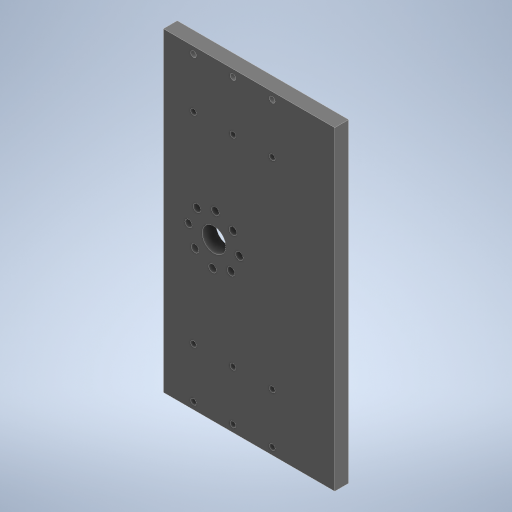
# Autodesk Inventor part: 12
Saved by Autodesk Inventor 2024.3 (Build 283343000, 343)
## iProperties
Created: 2024-09-08
Part Number: 12
Material: 아크릴, 선명
Document SubType Name: Modeling
Designer: 구지현
Density: 1.19 g/cm^3
Appearance: 회색
Mass: 66.4726 g
Surface Area: 217.278 cm^2
Volume: 55.8594 cm^3
Author: 구지현
Autodesk Inventor part; units mm, degrees
ref_plane "YZ Plane" through (0, 0, 0) normal (1, 0, 0) x (0, 1, 0)
ref_plane "XZ Plane" through (0, 0, 0) normal (0, 1, 0) x (-1, 0, 0)
ref_plane "XY Plane" through (0, 0, 0) normal (0, 0, 1) x (1, 0, 0)
ref_plane "작업 평면1" through (-11.501, -90.6951, 25.5) normal (0, 0, 1) x (0, 1, 0)
sketch "스케치1" plane through (-11.501, -90.6951, 25.5) normal (0, 0, 1) x (0, 1, 0)
  line L0 (-0.0049, 0) -> (27.5951, 0) projected
  line L1 (27.5951, 0) -> (27.5951, 6) projected
  line L2 (-0.0049, 6) -> (27.5951, 6) projected
  line L3 (-0.0049, 0) -> (-0.0049, 6) projected
  line L4 (127.3951, 6) -> (99.7951, 6) projected
  line L5 (99.7951, 6) -> (99.7951, 0) projected
  line L6 (127.3951, 0) -> (99.7951, 0) projected
  line L7 (127.3951, 6) -> (127.3951, 0) projected
  line L8 (99.8951, -54.101) -> (127.4951, -54.101) projected
  line L9 (127.4951, -54.101) -> (127.4951, -48.101) projected
  line L10 (99.8951, -48.101) -> (127.4951, -48.101) projected
  line L11 (99.8951, -54.101) -> (99.8951, -48.101) projected
  line L12 (27.4951, -48.101) -> (-0.1049, -48.101) projected
  line L13 (-0.1049, -48.101) -> (-0.1049, -54.101) projected
  line L14 (27.4951, -54.101) -> (-0.1049, -54.101) projected
  line L15 (27.4951, -48.101) -> (27.4951, -54.101) projected
  line L16 (-0.2463, -60.601) -> (-0.2463, -62.601) projected
  line L17 (-0.2463, -62.601) -> (1.1951, -62.601) projected
  line L18 (1.1951, -62.601) -> (1.1951, -92.601) projected
  line L19 (1.1951, -92.601) -> (-0.2463, -92.601) projected
  line L20 (-0.2463, -92.601) -> (-0.2463, -94.601) projected
  line L21 (-0.2463, -94.601) -> (6.0451, -94.601) projected
  line L22 (21.3451, -94.601) -> (6.0451, -94.601) projected
  line L23 (21.3451, -94.601) -> (27.6365, -94.601) projected
  line L24 (27.6365, -92.601) -> (27.6365, -94.601) projected
  line L25 (27.6365, -92.601) -> (26.1951, -92.601) projected
  line L26 (26.1951, -62.601) -> (26.1951, -92.601) projected
  line L27 (26.1951, -62.601) -> (27.6365, -62.601) projected
  line L28 (27.6365, -60.601) -> (27.6365, -62.601) projected
  line L29 (27.6365, -60.601) -> (26.6951, -60.601) projected
  line L30 (26.6951, -60.601) -> (26.6951, -59.101) projected
  line L31 (0.6951, -59.101) -> (26.6951, -59.101) projected
  line L32 (0.6951, -59.101) -> (0.6951, -60.601) projected
  line L33 (0.6951, -60.601) -> (-0.2463, -60.601) projected
  line L34 (35.6951, -14.501) -> (35.6951, -37.501) projected
  line L35 (35.6951, -14.501) -> (30.6951, -14.501) projected
  line L36 (30.6951, -14.501) -> (30.6951, -11.001) projected
  line L37 (28.6951, -11.001) -> (30.6951, -11.001) projected
  line L38 (28.6951, -11.001) -> (28.6951, -13.501) projected
  line L39 (28.6951, -13.501) -> (-1.3049, -13.501) projected
  line L40 (-1.3049, -13.501) -> (-1.3049, -11.001) projected
  line L41 (-1.3049, -11.001) -> (-3.3049, -11.001) projected
  line L42 (-3.3049, -11.001) -> (-3.3049, -16.751) projected
  line L43 (-5.8049, -16.751) -> (-3.3049, -16.751) projected
  spline S0 degree 3 poles (-5.8049, -16.751) (-6.0293, -16.751) (-6.2964, -16.7855) (-6.6655, -16.908) (-6.8416, -16.9972) (-7.0685, -17.1834) (-7.1685, -17.3017) (-7.2736, -17.5152) (-7.3049, -17.6421) (-7.3049, -17.751) knots -0.188065 -0.188065 -0.188065 -0.188065 -0.120738 -0.120738 -0.071394 -0.071394 -0.032672 -0.032672 0 0 0 0 projected
  line L44 (-7.3049, -34.251) -> (-7.3049, -17.751) projected
  spline S1 degree 3 poles (-7.3049, -34.251) (-7.3049, -34.3599) (-7.2736, -34.4868) (-7.1685, -34.7003) (-7.0685, -34.8186) (-6.8416, -35.0048) (-6.6655, -35.094) (-6.2964, -35.2165) (-6.0293, -35.251) (-5.8049, -35.251) knots 0 0 0 0 0.032672 0.032672 0.071394 0.071394 0.120738 0.120738 0.188065 0.188065 0.188065 0.188065 projected
  line L45 (-5.8049, -35.251) -> (-3.3049, -35.251) projected
  line L46 (-3.3049, -35.251) -> (-3.3049, -41.001) projected
  line L47 (-1.3049, -41.001) -> (-3.3049, -41.001) projected
  line L48 (-1.3049, -41.001) -> (-1.3049, -38.501) projected
  line L49 (28.6951, -38.501) -> (-1.3049, -38.501) projected
  line L50 (28.6951, -38.501) -> (28.6951, -41.001) projected
  line L51 (28.6951, -41.001) -> (30.6951, -41.001) projected
  line L52 (30.6951, -41.001) -> (30.6951, -37.501) projected
  line L53 (35.6951, -37.501) -> (30.6951, -37.501) projected
  line L54 (135.6951, -14.501) -> (135.6951, -37.501) projected
  line L55 (135.6951, -14.501) -> (130.6951, -14.501) projected
  line L56 (130.6951, -14.501) -> (130.6951, -11.001) projected
  line L57 (128.6951, -11.001) -> (130.6951, -11.001) projected
  line L58 (128.6951, -11.001) -> (128.6951, -13.501) projected
  line L59 (128.6951, -13.501) -> (98.6951, -13.501) projected
  line L60 (98.6951, -13.501) -> (98.6951, -11.001) projected
  line L61 (98.6951, -11.001) -> (96.6951, -11.001) projected
  line L62 (96.6951, -11.001) -> (96.6951, -16.751) projected
  line L63 (94.1951, -16.751) -> (96.6951, -16.751) projected
  spline S2 degree 3 poles (94.1951, -16.751) (93.9707, -16.751) (93.7036, -16.7855) (93.3345, -16.908) (93.1584, -16.9972) (92.9315, -17.1834) (92.8315, -17.3017) (92.7264, -17.5152) (92.6951, -17.6421) (92.6951, -17.751) knots -0.188065 -0.188065 -0.188065 -0.188065 -0.120738 -0.120738 -0.071394 -0.071394 -0.032672 -0.032672 0 0 0 0 projected
  line L64 (92.6951, -34.251) -> (92.6951, -17.751) projected
  spline S3 degree 3 poles (92.6951, -34.251) (92.6951, -34.3599) (92.7264, -34.4868) (92.8315, -34.7003) (92.9315, -34.8186) (93.1584, -35.0048) (93.3345, -35.094) (93.7036, -35.2165) (93.9707, -35.251) (94.1951, -35.251) knots 0 0 0 0 0.032672 0.032672 0.071394 0.071394 0.120738 0.120738 0.188065 0.188065 0.188065 0.188065 projected
  line L65 (94.1951, -35.251) -> (96.6951, -35.251) projected
  line L66 (96.6951, -35.251) -> (96.6951, -41.001) projected
  line L67 (98.6951, -41.001) -> (96.6951, -41.001) projected
  line L68 (98.6951, -41.001) -> (98.6951, -38.501) projected
  line L69 (128.6951, -38.501) -> (98.6951, -38.501) projected
  line L70 (128.6951, -38.501) -> (128.6951, -41.001) projected
  line L71 (128.6951, -41.001) -> (130.6951, -41.001) projected
  line L72 (130.6951, -41.001) -> (130.6951, -37.501) projected
  line L73 (135.6951, -37.501) -> (130.6951, -37.501) projected
  line L74 (99.7537, -60.601) -> (99.7537, -62.601) projected
  line L75 (99.7537, -62.601) -> (101.1951, -62.601) projected
  line L76 (101.1951, -62.601) -> (101.1951, -92.601) projected
  line L77 (101.1951, -92.601) -> (99.7537, -92.601) projected
  line L78 (99.7537, -92.601) -> (99.7537, -94.601) projected
  line L79 (99.7537, -94.601) -> (106.0451, -94.601) projected
  line L80 (121.3451, -94.601) -> (106.0451, -94.601) projected
  line L81 (121.3451, -94.601) -> (127.6365, -94.601) projected
  line L82 (127.6365, -92.601) -> (127.6365, -94.601) projected
  line L83 (127.6365, -92.601) -> (126.1951, -92.601) projected
  line L84 (126.1951, -62.601) -> (126.1951, -92.601) projected
  line L85 (126.1951, -62.601) -> (127.6365, -62.601) projected
  line L86 (127.6365, -60.601) -> (127.6365, -62.601) projected
  line L87 (127.6365, -60.601) -> (126.6951, -60.601) projected
  line L88 (126.6951, -60.601) -> (126.6951, -59.101) projected
  line L89 (100.6951, -59.101) -> (126.6951, -59.101) projected
  line L90 (100.6951, -59.101) -> (100.6951, -60.601) projected
  line L91 (100.6951, -60.601) -> (99.7537, -60.601) projected
  line L92 (21.3451, 6) -> (21.3451, 12)
  line L93 (1.1951, -62.601) -> (1.1951, 11.399)
  line L94 (-24.3049, -26.001) -> (-24.3049, -76.001) projected
  line L95 (-24.3049, -76.001) -> (-18.3049, -76.001) projected
  line L96 (-18.3049, -26.001) -> (-18.3049, -76.001) projected
  line L97 (-24.3049, -26.001) -> (-18.3049, -26.001) projected
  line L98 (145.6951, -26.001) -> (145.6951, -76.001) projected
  line L99 (145.6951, -76.001) -> (151.6951, -76.001) projected
  line L100 (151.6951, -26.001) -> (151.6951, -76.001) projected
  line L101 (145.6951, -26.001) -> (151.6951, -26.001) projected
  line L102 (-24.3049, -52.5323) -> (151.6951, -52.5323)
  line L103 (1.1951, 11.399) -> (-33.5056, 11.399)
  line L104 (1.1951, -62.601) -> (-24.3049, -62.601)
  line L105 (-24.3049, -62.601) -> (151.6951, -62.601)
  line L106 (151.6951, -62.601) -> (151.6951, 11.399)
  line L107 (151.6951, 11.399) -> (-24.3049, 11.399)
  line L108 (-24.3049, 11.399) -> (-24.3049, -62.601)
  circle A0 centre (-0.0049, 0) radius 1
  circle A1 centre (-0.0049, 6) radius 1
  circle A2 centre (27.5951, 6) radius 1
  circle A3 centre (27.5951, 0) radius 1
  circle A4 centre (99.7951, 0) radius 1
  circle A5 centre (99.7951, 6) radius 1
  circle A6 centre (127.3951, 6) radius 1
  circle A7 centre (127.3951, 0) radius 1
  circle A8 centre (99.8951, -54.101) radius 1
  circle A9 centre (99.8951, -48.101) radius 1
  circle A10 centre (127.4951, -48.101) radius 1
  circle A11 centre (127.6365, -54.101) radius 1
  circle A12 centre (27.4951, -54.101) radius 1
  circle A13 centre (27.5951, -48.101) radius 1
  circle A14 centre (-0.1049, -48.101) radius 1
  circle A15 centre (-0.1049, -54.101) radius 1
  point P0 (90.6951, -11.501)
  point P1 (99.8951, -49.101)
  point P2 (100.8951, -48.101)
  point P3 (126.4951, -48.101)
  point P4 (127.4951, -49.101)
  point P5 (127.4951, -53.1111)
  point P6 (126.6365, -54.101)
  point P7 (100.8951, -54.101)
  point P8 (99.8951, -53.101)
  point P9 (126.3951, 0)
  point P10 (100.7951, 0)
  point P11 (99.7951, 1)
  point P12 (99.7951, 5)
  point P13 (100.7951, 6)
  point P14 (126.3951, 6)
  point P15 (127.3951, 5)
  point P16 (127.3951, 1)
  point P17 (26.5951, 6)
  point P18 (27.5951, 5)
  point P19 (27.5951, 1)
  point P20 (26.5951, 0)
  point P21 (0.9951, 0)
  point P22 (-0.0049, 1)
  point P23 (-0.0049, 5)
  point P24 (0.9951, 6)
  point P25 (26.5951, -48.101)
  point P26 (27.4951, -49.096)
  point P27 (27.4951, -53.101)
  point P28 (26.4951, -54.101)
  point P29 (0.8951, -54.101)
  point P30 (-0.1049, -53.101)
  point P31 (-0.1049, -49.101)
  point P32 (0.8951, -48.101)
  point P33 (-0.2463, -62.601)
  point P34 (1.1951, -62.601)
  point P35 (99.7537, -62.601)
  point P36 (101.1951, -62.601)
  point P37 (126.1951, -62.601)
  point P38 (127.6365, -62.601)
  point P39 (151.6951, -62.601)
  point P40 (1.1951, 11.399)
  point P41 (-24.3049, 11.399)
  dimension "d0" = 6
  dimension "d1" = 74
  dimension "d2" = 2
  dimension "d3" = 2
  dimension "d4" = 2
  dimension "d5" = 2
  dimension "d6" = 2
  dimension "d7" = 2
  dimension "d8" = 2
  dimension "d9" = 2
  dimension "d10" = 2
  dimension "d11" = 2
  dimension "d12" = 2
  dimension "d13" = 2
  dimension "d14" = 2
  dimension "d15" = 2
  dimension "d16" = 2
  dimension "d17" = 2
  constraints: 18 end point, 16 centre point, 14 coincident, 4 point on line, 3 perpendicular, 2 horizontal, 2 parallel, 2 vertical
  measures "d0" distance of L92.start L92.end
  measures "d1" distance of L17.end L93.end
  measures "d2" diameter of A0
  measures "d3" diameter of A1
  measures "d4" diameter of A2
  measures "d5" diameter of A3
  measures "d6" diameter of A4
  measures "d7" diameter of A5
  measures "d8" diameter of A6
  measures "d9" diameter of A7
  measures "d10" diameter of A8
  measures "d11" diameter of A9
  measures "d12" diameter of A10
  measures "d13" diameter of A11
  measures "d14" diameter of A12
  measures "d15" diameter of A13
  measures "d16" diameter of A14
  measures "d17" diameter of A15
extrude "돌출1" add sketch "스케치1" along normal blind 6 contours L3 A0 L0 | L0 A0 L3 | A0 L3 A1 L2 L93 L0 | L0 L93 L39 L40 L41 L42 L43 S0 L44 S1 L45 L46 L47 L48 L49 L12 A14 L13 L102 L96 L97 L108 L103 L2 A1 L3 A0 | L93 L2 A2 L1 A3 L0 | L0 A3 L1 A2 L2 L92 L107 L106 L101 L98 L102 L9 A10 L10 A9 L11 L15 A13 L12 L93 L49 L50 L51 L52 L53 L34 L35 L36 L37 L38 L39 | A1 L2 L3 | L3 L2 A1 | A3 L1 L0 | L0 L1 A3 | L93 L49 L48 L47 L46 L45 S1 L44 S0 L43 L42 L41 L40 L39 | L39 L38 L37 L36 L35 L34 L53 L52 L51 L50 L49 L93 | L93 L107 L92 L2 | A2 L2 L1 | L1 L2 A2 | L93 L102 L13 A14 L12 | L12 A13 L15 L102 L93 | A13 L15 L12 | L12 L15 A13 | A14 L13 L12 | L12 L13 A14 | L102 L15 A12 L14 L93 | L93 L14 A15 L13 L102 | L97 L96 L102 L94 | L93 L31 L32 L33 L16 L104 L96 L102 L13 A15 L14 | L14 A12 L15 L102 L11 A8 L8 A11 L9 L98 L105 L86 L87 L88 L89 L90 L91 L74 L28 L29 L30 L31 L93 | L100 L102 L98 L101 | L102 L96 L104 L94 | A12 L15 L14 | L14 L15 A12 | A15 L13 L14 | L14 L13 A15 | L93 L17 L16 L33 L32 L31 | L31 L30 L29 L28 L27 L105 L93 | L102 L9 A11 L8 A8 L11 | L11 A9 L10 A10 L9 L102 | L100 L105 L98 L102 | A8 L8 L11 | L11 L8 A8 | A9 L10 L11 | L11 L10 A9 | A11 L8 L9 | L9 L8 A11 | A10 L10 L9 | L9 L10 A10 | L85 L105 L75 L74 L91 L90 L89 L88 L87 L86 | A5 L5 L4 | L4 L5 A5 | L4 A6 L7 A7 L6 A4 L5 A5 | A6 L7 L4 | L4 L7 A6 | A4 L6 L5 | L5 L6 A4 | A7 L6 L7 | L7 L6 A7 | L54 L73 L72 L71 L70 L69 L68 L67 L66 L65 S3 L64 S2 L63 L62 L61 L60 L59 L58 L57 L56 L55
sketch "스케치3" plane through (-11.501, -90.6951, 31.5) normal (0, 0, 1) x (1, 0, 0)
  line L0 (-11.399, 151.6951) -> (-11.399, -24.3049) projected
  line L1 (-11.399, 151.6951) -> (-11.399, 63.6951)
  line L2 (62.601, -24.3049) -> (62.601, 151.6951) projected
  line L3 (62.601, 151.6951) -> (-11.399, 151.6951) projected
  line L4 (-11.399, 151.6951) -> (-11.399, -24.3049) projected
  line L5 (-11.399, -24.3049) -> (62.601, -24.3049) projected
  line L6 (-11.399, 63.6951) -> (62.601, 63.6951)
  circle A0 centre (-0.5531, 64.2887) radius 1.55 projected
  circle A1 centre (11.0245, 74.6791) radius 1.55 projected
  circle A2 centre (21.4149, 63.1016) radius 1.55 projected
  circle A3 centre (9.8373, 52.7111) radius 1.55 projected
  circle A4 centre (10.4309, 63.6951) radius 5 projected
  circle A5 centre (10.4309, 63.6951) radius 13.9 projected
  circle A6 centre (17.778, 55.5086) radius 1.55 projected
  circle A7 centre (18.6175, 71.0422) radius 1.55 projected
  circle A8 centre (3.0838, 71.8817) radius 1.55 projected
  circle A9 centre (2.2443, 56.348) radius 1.55 projected
  circle A10 centre (3.0838, 71.8817) radius 1.65
  circle A11 centre (-0.5531, 64.2887) radius 1.65
  circle A12 centre (2.2443, 56.348) radius 1.65
  circle A13 centre (9.8373, 52.7111) radius 1.65
  circle A14 centre (17.778, 55.5086) radius 1.65
  circle A15 centre (21.4149, 63.1016) radius 1.65
  circle A16 centre (18.6175, 71.0422) radius 1.65
  circle A17 centre (11.0245, 74.6791) radius 1.65
  circle A18 centre (10.4309, 63.6951) radius 5.1
  point P0 (11.501, 90.6951)
  dimension "d32" = 88
  dimension "d33" = 0.1
  dimension "d34" = 0.1
  dimension "d35" = 0.1
  dimension "d36" = 0.1
  dimension "d37" = 0.1
  dimension "d38" = 0.1
  dimension "d39" = 0.1
  dimension "d40" = 0.1
  dimension "d41" = 0.1
  constraints: 9 centre point, 4 end point, 2 midpoint
  measures "d32" distance of L0.start L1.end
  measures "d33" radial gap between concentric circles of A8 A10
  measures "d34" radial gap between concentric circles of A0 A11
  measures "d35" radial gap between concentric circles of A9 A12
  measures "d36" radial gap between concentric circles of A3 A13
  measures "d37" radial gap between concentric circles of A6 A14
  measures "d38" radial gap between concentric circles of A2 A15
  measures "d39" radial gap between concentric circles of A7 A16
  measures "d40" radial gap between concentric circles of A1 A17
  measures "d41" radial gap between concentric circles of A4 A18
extrude "돌출3" cut sketch "스케치3" against normal blind 10 contours A0 L6 | L6 A0 | A15 L6 A2 | L6 A2 A15 | A18 L6 A4 | L6 A4 A18 | A2 L6 | L6 A2 | A4 L6 | L6 A4 | A1 | A3 | A6 | A7 | A8 | A9 | A10 | A12 | A13 | A14 | A16 | A17
sketch "스케치8" plane through (-11.501, -90.6951, 31.5) normal (0, 0, 1) x (1, 0, 0)
  circle A0 centre (-0.5531, 64.2887) radius 1.55 projected
  circle A1 centre (17.778, 55.5086) radius 1.65 projected
  circle A2 centre (21.4149, 63.1016) radius 1.65 projected
  circle A3 centre (10.4309, 63.6951) radius 5.1 projected
  circle A4 centre (3.0838, 71.8817) radius 1.65 projected
  circle A5 centre (9.8373, 52.7111) radius 1.65 projected
  circle A6 centre (18.6175, 71.0422) radius 1.65 projected
  circle A7 centre (2.2443, 56.348) radius 1.65 projected
  circle A8 centre (11.0245, 74.6791) radius 1.65 projected
  line L0 (62.601, -24.3049) -> (62.601, 151.6951) projected
  line L1 (62.601, 151.6951) -> (-11.399, 151.6951) projected
  line L2 (-11.399, 151.6951) -> (-11.399, -24.3049) projected
  line L3 (-11.399, -24.3049) -> (62.601, -24.3049) projected
  line L4 (-11.399, -24.3049) -> (-11.399, -4.3049)
  line L5 (-11.399, 151.6951) -> (-11.399, -24.3049) projected
  line L6 (-11.399, 151.6951) -> (-11.399, 131.6951)
  line L7 (62.601, -24.3049) -> (62.601, 151.6951) projected
  line L8 (62.601, 151.6951) -> (-11.399, 151.6951)
  line L9 (-11.399, 151.6951) -> (-11.399, 131.6951)
  line L10 (-11.399, 131.6951) -> (62.601, 131.6951)
  line L11 (62.601, 131.6951) -> (62.601, 151.6951)
  line L12 (62.601, -24.3049) -> (-11.399, -24.3049)
  line L13 (-11.399, -24.3049) -> (-11.399, -4.3049)
  line L14 (-11.399, -4.3049) -> (62.601, -4.3049)
  line L15 (62.601, -4.3049) -> (62.601, -24.3049)
  line L16 (10.4309, 63.6951) -> (10.4309, 3.6951)
  line L17 (10.4309, 63.6951) -> (10.4309, 123.6951)
  line L18 (10.4309, 123.6951) -> (10.4309, 131.6951)
  line L19 (10.4309, 3.6951) -> (10.4309, -4.3049)
  point P0 (11.501, 90.6951)
  point P1 (-11.399, 131.6951)
  point P2 (62.601, 131.6951)
  point P3 (62.601, -4.3049)
  point P4 (-11.399, -4.3049)
  dimension "d55" = 20
  dimension "d56" = 20
  dimension "d59" = 60
  dimension "d60" = 60
  constraints: 28 end point, 5 point on line, 4 parallel, 3 perpendicular, 2 horizontal, 2 vertical
  measures "d55" distance of L2.end L4.end
  measures "d56" distance of L1.end L6.end
  measures "d59" distance of L16.start L16.end
  measures "d60" distance of L16.start L17.end
extrude "돌출8" cut sketch "스케치8" against normal blind 6 contours L10 L2 L1 L0 | L14 L0 L3 L2
sketch "스케치9" plane through (-11.501, -90.6951, 31.5) normal (0, 0, 1) x (1, 0, 0)
  line L0 (42.702, -4.3049) -> (42.702, 23.2951) projected
  line L1 (-5.399, -4.3049) -> (42.702, -4.3049) projected
  line L2 (-5.399, 23.2951) -> (-5.399, -4.3049) projected
  line L3 (42.702, 23.2951) -> (-5.399, 23.2951) projected
  line L4 (42.702, 104.0951) -> (42.702, 131.6951) projected
  line L5 (-5.399, 104.0951) -> (42.702, 104.0951) projected
  line L6 (-5.399, 131.6951) -> (-5.399, 104.0951) projected
  line L7 (42.702, 131.6951) -> (-5.399, 131.6951) projected
  line L8 (-5.399, -4.3049) -> (-5.399, -1.3049)
  line L9 (-5.399, -1.3049) -> (1.601, -1.3049)
  circle A0 centre (1.601, -1.3049) radius 1.25
  line L10 (1.601, -1.3049) -> (18.601, -1.3049)
  line L11 (18.601, -1.3049) -> (35.601, -1.3049)
  line L12 (35.601, -1.3049) -> (42.601, -1.3049)
  circle A1 centre (18.601, -1.3049) radius 1.25
  circle A2 centre (35.601, -1.3049) radius 1.25
  line L13 (-5.399, 23.2951) -> (-5.399, 20.2951)
  line L14 (-5.399, 23.2951) -> (-2.399, 23.2951) construction
  circle A3 centre (1.601, 20.2951) radius 1.25
  circle A4 centre (18.601, 20.2951) radius 1.25
  circle A5 centre (35.601, 20.2951) radius 1.25
  line L15 (-5.399, 104.0951) -> (-5.399, 107.0951)
  line L16 (-5.399, 107.0951) -> (1.601, 107.0951)
  line L17 (1.601, 107.0951) -> (18.601, 107.0951)
  line L18 (18.601, 107.0951) -> (35.601, 107.0951)
  line L19 (35.601, 107.0951) -> (42.601, 107.0951)
  circle A6 centre (1.601, 107.0951) radius 1.25
  circle A7 centre (18.601, 107.0951) radius 1.25
  circle A8 centre (35.601, 107.0951) radius 1.25
  line L20 (-5.399, 131.6951) -> (-5.399, 128.6951)
  circle A9 centre (1.601, 128.6951) radius 1.25
  circle A10 centre (18.601, 128.6951) radius 1.25
  circle A11 centre (35.601, 128.6951) radius 1.25
  line L21 (35.601, 107.0951) -> (35.601, 128.6951)
  line L22 (18.601, 107.0951) -> (18.601, 128.6951)
  line L23 (1.601, 107.0951) -> (1.601, 128.6951)
  line L24 (1.601, -1.3049) -> (1.601, 20.2951)
  line L25 (18.601, -1.3049) -> (18.601, 20.2951)
  line L26 (35.601, -1.3049) -> (35.601, 20.2951)
  circle A12 centre (1.601, 107.0951) radius 1.25 projected
  circle A13 centre (35.601, 128.6951) radius 1.25 projected
  circle A14 centre (18.601, 107.0951) radius 1.25 projected
  circle A15 centre (1.601, 128.6951) radius 1.25 projected
  circle A16 centre (18.601, 128.6951) radius 1.25 projected
  circle A17 centre (35.601, 107.0951) radius 1.25 projected
  circle A18 centre (1.601, -1.3049) radius 1.25 projected
  circle A19 centre (35.601, 20.2951) radius 1.25 projected
  circle A20 centre (18.601, -1.3049) radius 1.25 projected
  circle A21 centre (1.601, 20.2951) radius 1.25 projected
  circle A22 centre (18.601, 20.2951) radius 1.25 projected
  circle A23 centre (35.601, -1.3049) radius 1.25 projected
  dimension "d63" = 3
  dimension "d64" = 7
  dimension "d65" = 2.5
  dimension "d66" = 17
  dimension "d67" = 17
  dimension "d68" = 7
  dimension "d69" = 2.5
  dimension "d70" = 2.5
  dimension "d71" = 3
  dimension "d72" = 90
  dimension "d73" = 2.5
  dimension "d74" = 2.5
  dimension "d75" = 2.5
  dimension "d76" = 3
  dimension "d77" = 7
  dimension "d78" = 17
  dimension "d79" = 17
  dimension "d80" = 7
  dimension "d81" = 2.5
  dimension "d82" = 2.5
  dimension "d83" = 2.5
  dimension "d84" = 3
  dimension "d85" = 2.5
  dimension "d86" = 2.5
  dimension "d87" = 2.5
  constraints: 38 end point, 12 centre point, 6 coincident, 6 point on line, 5 perpendicular, 4 horizontal, 4 vertical, 1 collinear
  measures "d63" distance of L1.start L8.end
  measures "d64" distance of L8.end L9.end
  measures "d65" diameter of A0
  measures "d66" distance of L10.start L10.end
  measures "d67" distance of L10.end L11.end
  measures "d68" distance of L11.end L12.end
  measures "d69" diameter of A1
  measures "d70" diameter of A2
  measures "d71" distance of L2.start L13.end
  measures "d72" angle of L13 L14
  measures "d73" diameter of A3
  measures "d74" diameter of A4
  measures "d75" diameter of A5
  measures "d76" distance of L5.start L15.end
  measures "d77" distance of L15.end L16.end
  measures "d78" distance of L16.end L17.end
  measures "d79" distance of L17.end L18.end
  measures "d80" distance of L18.end L19.end
  measures "d81" diameter of A6
  measures "d82" diameter of A7
  measures "d83" diameter of A8
  measures "d84" distance of L6.start L20.end
  measures "d85" diameter of A9
  measures "d86" diameter of A10
  measures "d87" diameter of A11
extrude "돌출9" cut sketch "스케치9" against normal blind 20 contours A3 | A4 | A5 | A2 L26 L11 | L11 L12 A2 | A1 L25 L10 | L10 L11 A1 | A0 L24 L9 | L9 L10 A0 | L24 A0 L10 | L25 A1 L11 | L26 A2 L12 | A9 | A10 | A11 | A8 L21 L18 | L18 L19 A8 | A7 L22 L17 | L17 L18 A7 | A6 L23 L16 | L16 L17 A6 | L23 A6 L17 | L22 A7 L18 | L21 A8 L19
